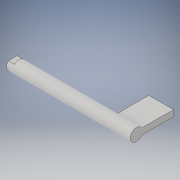
# Autodesk Inventor part: StressTestPart
Saved by Autodesk Inventor 2017 (Build 210142000, 142)
## iProperties
Created: 2018-03-21
Part Number: StressTestPart
Material: Generic
Document SubType Name: Modeling
Designer: User
Density: 1 g/cm^3
Appearance: Default
Mass: 21.1777 g
Surface Area: 73.691 cm^2
Volume: 21.1777 cm^3
Author: User
Autodesk Inventor part; units mm, degrees
ref_plane "YZ Plane" through (0, 0, 0) normal (1, 0, 0) x (0, 1, 0)
ref_plane "XZ Plane" through (0, 0, 0) normal (0, 1, 0) x (-1, 0, 0)
ref_plane "XY Plane" through (0, 0, 0) normal (0, 0, 1) x (1, 0, 0)
sketch "Sketch1" plane through (0, 0, 0) normal (1, 0, 0) x (0, 1, 0)
  circle A0 centre (0, 0) radius 6.35
  dimension "d0" = 12.7
  constraints: 1 centre point, 1 coincident
  measures "d0" diameter of A0
extrude "Extrusion1" add sketch "Sketch1" along normal blind 127
sketch "Sketch2" plane through (127, 0, 0) normal (1, 0, 0) x (0, 0, -1)
  circle A0 centre (0, 0) radius 6.35 projected
  line L0 (0, 3.175) -> (38.1, 3.175)
  line L1 (38.1, 3.175) -> (38.1, -3.175)
  line L2 (38.1, -3.175) -> (0, -3.175)
  line L3 (0, -3.175) -> (0, 3.175)
  dimension "d3" = 12.7
  dimension "d4" = 6.35
  dimension "d5" = 3.175
  dimension "d6" = 38.1
  dimension "d7" = 0
  constraints: 8 end point, 2 parallel, 1 horizontal, 1 perpendicular
  measures "d3" diameter of A0
  measures "d4" distance of L0.end L1.end
  measures "d5" distance from line of L0 point (0, 0)
  measures "d6" distance of L0.start L0.end
  measures "d7" distance from line of point (0, 0) L3
extrude "Extrusion2" add sketch "Sketch2" against normal blind 25.4 contours A0 L2 L3 L0 | A0 L0 L1 L2 picked at (2.1167, 0)
sketch "Sketch3" plane through (0, 0, 0) normal (-1, 0, 0) x (0, 0, 1)
  circle A0 centre (0, 0) radius 6.35 projected
  circle A1 centre (0, 0) radius 6.35 projected
  line L0 (-4.5348, 4.445) -> (4.5348, 4.445)
  line L1 (-5.4993, 3.175) -> (-38.1, 3.175) projected
  dimension "d10" = 4.445
  constraints: 4 point on circle, 2 end point, 1 parallel
  measures "d10" distance from line of L0 point (0, 0)
extrude "Extrusion3" cut sketch "Sketch3" against normal blind 6.35 contours L0 A0 picked at (-0.24, 5.0664)
body "Solid1"
